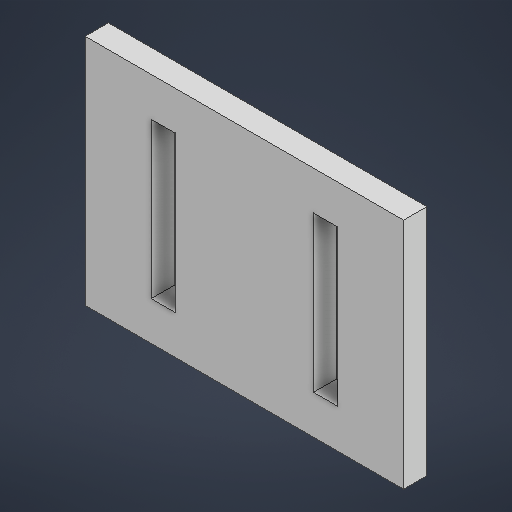
# Autodesk Inventor part: Moving_rail
Saved by Autodesk Inventor 2027 (Build 310192000, 192)
## iProperties
Created: 2026-05-09
Part Number: Moving_rail
Material: Generic
Document SubType Name: Modeling
Designer: alexy
Density: 1 g/cm^3
Appearance: Default
Author: alexy
Autodesk Inventor part; units mm, degrees
ref_plane "YZ Plane" through (0, 0, 0) normal (1, 0, 0) x (0, 1, 0)
ref_plane "XZ Plane" through (0, 0, 0) normal (0, 1, 0) x (-1, 0, 0)
ref_plane "XY Plane" through (0, 0, 0) normal (0, 0, 1) x (1, 0, 0)
sketch "Sketch1" plane through (0, 0, 0) normal (0, 0, 1) x (1, 0, 0)
  line L0 (0, 0) -> (41, 0)
  line L1 (41, 0) -> (41, 30)
  line L2 (41, 30) -> (0, 30)
  line L3 (0, 30) -> (0, 0)
  line L4 (29.4, 25) -> (32.5, 25)
  line L5 (32.5, 25) -> (32.5, 5)
  line L6 (32.5, 5) -> (29.4, 5)
  line L7 (29.4, 5) -> (29.4, 25)
  line L8 (8.5, 25) -> (11.6, 25)
  line L9 (11.6, 25) -> (11.6, 5)
  line L10 (11.6, 5) -> (8.5, 5)
  line L11 (8.5, 5) -> (8.5, 25)
  point P0 (8.5, 15)
  point P1 (0, 15)
  point P2 (29.4, 15)
  point P3 (10.05, 5)
  point P4 (20.5, 30)
  dimension "d0" = 41
  dimension "d1" = 30
  dimension "d2" = 3.1
  dimension "d3" = 3.1
  dimension "d4" = 24
  dimension "d6" = 10
  dimension "d7" = 8.9
  constraints: 24 end point, 6 parallel, 5 midpoint, 3 horizontal, 3 perpendicular, 2 horizontal alignment, 2 point on line
  measures "d0" distance of L2.end L1.end
  measures "d1" distance of L0.end L1.end
  measures "d2" distance of L5.end L6.end
  measures "d3" distance of L9.end L10.end
  measures "d4" distance between parallel lines of L11 L5
  measures "d6" vertical distance of point (8.5, 15) point (10.05, 5)
  measures "d7" distance from line of L9 point (20.5, 30)
extrude "Extrusion1" add sketch "Sketch1" along normal blind 3
body "Solid1"
